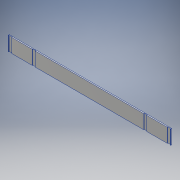
# Autodesk Inventor part: 앞판_중간
Saved by Autodesk Inventor 2017 (Build 210142000, 142)
## iProperties
Part Number: 앞판_중간
Material: 알루미늄 6061
Document SubType Name: Modeling
Designer: minom
Density: 2.7 g/cm^3
Appearance: 알루미늄 - 평지
Mass: 37.692 g
Surface Area: 159.168 cm^2
Volume: 13.96 cm^3
Author: minom
Autodesk Inventor part; units mm, degrees
ref_plane "YZ Plane" through (0, 0, 0) normal (1, 0, 0) x (0, 1, 0)
ref_plane "XZ Plane" through (0, 0, 0) normal (0, 1, 0) x (-1, 0, 0)
ref_plane "XY Plane" through (0, 0, 0) normal (0, 0, 1) x (1, 0, 0)
sketch "스케치1" plane through (0, 0, 0) normal (0, 1, 0) x (-1, 0, 0)
  line L0 (197, 1) -> (-93, 1)
  line L1 (-93, 1) -> (-93, 26)
  line L2 (-93, 26) -> (197, 26)
  line L3 (197, 26) -> (197, 1)
  point P0 (0, 0)
  dimension "d0" = 290
  dimension "d1" = 25
  constraints: 8 end point, 2 parallel, 1 horizontal, 1 perpendicular
  measures "d0" distance of L1.end L2.end
  measures "d1" distance of L0.end L1.end
extrude "돌출1" add sketch "스케치1" along normal blind 2
sketch "스케치2" plane through (0, 0, 0) normal (0, -1, 0) x (1, 0, 0)
  line L0 (-197, 26) -> (93, 26) projected
  line L1 (93, 1) -> (-197, 1) projected
  line L2 (-154, 26) -> (-148.6, 26)
  line L3 (-148.6, 26) -> (-148.6, 1)
  line L4 (-148.6, 1) -> (-154, 1)
  line L5 (-154, 1) -> (-154, 26)
  line L6 (44.6, 26) -> (50, 26)
  line L7 (50, 26) -> (50, 1)
  line L8 (50, 1) -> (44.6, 1)
  line L9 (44.6, 1) -> (44.6, 26)
  line L10 (-197, 26) -> (-197, 1) projected
  line L11 (93, 1) -> (93, 26) projected
  point P0 (0, 0)
  dimension "d4" = 5.4
  dimension "d5" = 5.4
  dimension "d6" = 43
  dimension "d7" = 43
  constraints: 16 end point, 4 parallel, 2 horizontal, 2 perpendicular, 2 point on line, 3 other
  measures "d4" distance of L3.end L4.end
  measures "d5" distance of L7.end L8.end
  measures "d6" distance between parallel lines of L5 L10
  measures "d7" distance between parallel lines of L11 L7
extrude "돌출2" cut sketch "스케치2" against normal blind 1 contours L0 L3 L1 L5 | L0 L7 L1 L9
sketch "스케치3" plane through (0, 0, 0) normal (0, -1, 0) x (1, 0, 0)
  line L0 (50, 26) -> (50, 1) projected
  line L1 (50, 1) -> (93, 1) projected
  line L2 (93, 1) -> (93, 26) projected
  line L3 (93, 26) -> (50, 26) projected
  line L4 (-154, 1) -> (-154, 26) projected
  line L5 (-154, 26) -> (-197, 26) projected
  line L6 (-197, 26) -> (-197, 1) projected
  line L7 (-197, 1) -> (-154, 1) projected
  line L8 (50, 1) -> (93, 1) projected
  line L9 (92, 1) -> (92, 26)
  line L10 (86.6, 1) -> (86.6, 26)
  line L11 (-196, 1) -> (-196, 26)
  line L12 (93, 1) -> (-197, 1) projected
  line L13 (-190.6, 1) -> (-190.6, 26)
  point P0 (0, 0)
  dimension "d10" = 1
  dimension "d11" = 5.4
  dimension "d12" = 1
  dimension "d13" = 5.4
  constraints: 8 end point, 8 point on line, 3 perpendicular, 1 vertical
  measures "d10" distance between parallel lines of L6 L11
  measures "d11" distance between parallel lines of L11 L13
  measures "d12" distance between parallel lines of L2 L9
  measures "d13" distance between parallel lines of L9 L10
extrude "돌출3" cut sketch "스케치3" against normal blind 1 contours L3 L9 L1 L10 | L7 L11 L5 L13
